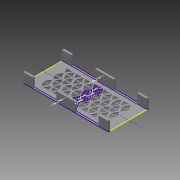
# Autodesk Inventor part: BandSide
Saved by Autodesk Inventor 2014 SP1 (Build 180222100, 222)
## iProperties
Created: 2015-03-16
Part Number: BandSide
Material: Generic
Document SubType Name: Modeling
Designer: Erin
Density: 1 g/cm^3
Appearance: Default
Author: Erin
Autodesk Inventor part; units mm, degrees
ref_plane "YZ Plane" through (0, 0, 0) normal (1, 0, 0) x (0, 1, 0)
ref_plane "XZ Plane" through (0, 0, 0) normal (0, 1, 0) x (-1, 0, 0)
ref_plane "XY Plane" through (0, 0, 0) normal (0, 0, 1) x (1, 0, 0)
sketch "Block1" plane through (0, 0, 0) normal (0, 0, 1) x (1, 0, 0)
  line L0 (-5.6547, 8.5) -> (0.3453, 8.5)
  line L1 (0.3453, 8.5) -> (-2.6547, 3.3038)
  line L2 (-2.6547, 3.3038) -> (-5.6547, 8.5)
  line L3 (5.6547, 3.3038) -> (-0.3453, 3.3038)
  line L4 (-0.3453, 3.3038) -> (2.6547, 8.5)
  line L5 (2.6547, 8.5) -> (5.6547, 3.3038)
  line L6 (-5.6547, 8.5) -> (5.6547, 8.5) construction
  line L7 (5.6547, 8.5) -> (5.6547, 3.3038) construction
  line L8 (5.6547, 3.3038) -> (-5.6547, 3.3038) construction
  line L9 (-5.6547, 3.3038) -> (-5.6547, 8.5) construction
  line L10 (0, 8.5) -> (0, 3.3038) construction
  line L11 (5.6547, 5.9019) -> (-5.6547, 5.9019) construction
  point P0 (0.0717, 5.9721)
  point P1 (-2.6547, 6.7679)
  point P2 (2.6547, 5.0359)
  dimension "d11" = 6
  dimension "d12" = 6
  dimension "d13" = 2
  measures "d11" distance of L0.start L0.end
  measures "d12" distance of L3.start L3.end
  measures "d13" distance between parallel lines of L1 L4
sketch "Sketch1" plane through (0, 0, 0) normal (0, 0, 1) x (1, 0, 0)
  line L0 (-45, 21.5) -> (45, 21.5)
  line L1 (45, 21.5) -> (45, -21.5)
  line L2 (45, -21.5) -> (-45, -21.5)
  line L3 (-45, -21.5) -> (-45, 21.5)
  line L4 (-45, 21.5) -> (-51, 21.5)
  line L5 (-51, 21.5) -> (-51, -21.5)
  line L6 (-51, -21.5) -> (-45, -21.5)
  line L7 (-45, -21.5) -> (-45, 21.5)
  line L8 (-51, 21.5) -> (-91, 21.5)
  line L9 (-91, 21.5) -> (-91, -21.5)
  line L10 (-91, -21.5) -> (-51, -21.5)
  line L11 (-51, -21.5) -> (-51, 21.5)
  line L12 (-91, 21.5) -> (-97, 21.5)
  line L13 (-97, 21.5) -> (-97, -21.5)
  line L14 (-97, -21.5) -> (-91, -21.5)
  line L15 (-91, -21.5) -> (-91, 21.5)
  line L16 (-174.2812, 12.5) -> (-97, 12.5) construction
  line L17 (-97, 12.5) -> (-97, -12.5) construction
  line L18 (-97, -12.5) -> (-174.2812, -12.5) construction
  line L19 (-174.2812, -12.5) -> (-174.2812, 12.5) construction
  line L20 (-127, 31.5284) -> (-127, -21.68) construction
  line L21 (-97, 21.5) -> (-127, 12.5)
  line L22 (-97, -21.5) -> (-127, -12.5)
  line L23 (-127, 12.5) -> (-127, -12.5)
  line L24 (-127, 10) -> (-142, 10)
  line L25 (-142, 10) -> (-142, -10)
  line L26 (-142, -10) -> (-127, -10)
  line L27 (-127, -10) -> (-127, 10)
  point P0 (0, 0)
  point P1 (-45, 0)
  point P2 (0, 21.5)
  point P3 (-97, 0)
  point P4 (-142, 0)
  dimension "d0" = 90
  dimension "d1" = 43
  dimension "d2" = 6
  dimension "d3" = 40
  dimension "d4" = 6
  dimension "d5" = 25
  dimension "d6" = 30
  dimension "d7" = 15
  dimension "d8" = 20
  constraints: 56 end point, 13 parallel, 7 perpendicular, 6 horizontal, 5 point on line, 4 collinear, 4 midpoint, 3 horizontal alignment, 1 vertical alignment
  measures "d0" distance of L1.end L2.end
  measures "d1" distance of L0.end L1.end
  measures "d2" distance of L6.end L5.end
  measures "d3" distance of L10.end L9.end
  measures "d4" distance of L14.end L13.end
  measures "d5" distance of L18.end L16.start
  measures "d6" distance between parallel lines of L20 L13
  measures "d7" distance of L26.end L25.end
  measures "d8" distance of L25.end L24.end
extrude "Extrusion1" add sketch "Sketch1" along normal blind 0.6 contours L0 L1 L2 L3
sketch "Sketch2" plane through (0, 0, 0.6) normal (0, 0, 1) x (1, 0, 0)
  line L0 (-45, 21.5) -> (-45, -21.5) projected
  line L1 (-45, -21.5) -> (45, -21.5) projected
  line L2 (45, -21.5) -> (45, 21.5) projected
  line L3 (45, 21.5) -> (-45, 21.5) projected
  line L4 (-45, -19.5) -> (45, -19.5)
  line L5 (45, 19.5) -> (-45, 19.5)
  line L6 (-45, 19.5) -> (-45, 21.5)
  line L7 (-45, 21.5) -> (45, 21.5)
  line L8 (45, 21.5) -> (45, 19.5)
  line L9 (-45, -19.5) -> (-45, -21.5)
  line L10 (-45, -21.5) -> (45, -21.5)
  line L11 (45, -21.5) -> (45, -19.5)
  line L12 (0, 33.8236) -> (0, -26.1738) construction
  line L13 (-56.1802, 0) -> (59.4276, 0) construction
  line L14 (-5.6547, 14.9904) -> (0.3453, 14.9904)
  line L15 (0.3453, 14.9904) -> (-2.6547, 9.7942)
  line L16 (-2.6547, 9.7942) -> (-5.6547, 14.9904)
  line L17 (5.6547, 9.7942) -> (-0.3453, 9.7942)
  line L18 (-0.3453, 9.7942) -> (2.6547, 14.9904)
  line L19 (2.6547, 14.9904) -> (5.6547, 9.7942)
  line L20 (-5.6547, 14.9904) -> (5.6547, 14.9904) construction
  line L21 (5.6547, 14.9904) -> (5.6547, 9.7942) construction
  line L22 (5.6547, 9.7942) -> (-5.6547, 9.7942) construction
  line L23 (-5.6547, 9.7942) -> (-5.6547, 14.9904) construction
  line L24 (0, 14.9904) -> (0, 9.7942) construction
  line L25 (5.6547, 12.3923) -> (-5.6547, 12.3923) construction
  line L26 (5.6547, 8.7942) -> (-0.3453, 8.7942)
  line L27 (-0.3453, 8.7942) -> (2.6547, 3.5981)
  line L28 (2.6547, 3.5981) -> (5.6547, 8.7942)
  line L29 (-5.6547, 3.5981) -> (0.3453, 3.5981)
  line L30 (0.3453, 3.5981) -> (-2.6547, 8.7942)
  line L31 (-2.6547, 8.7942) -> (-5.6547, 3.5981)
  line L32 (5.6547, 8.7942) -> (-5.6547, 8.7942) construction
  line L33 (-5.6547, 8.7942) -> (-5.6547, 3.5981) construction
  line L34 (-5.6547, 3.5981) -> (5.6547, 3.5981) construction
  line L35 (5.6547, 3.5981) -> (5.6547, 8.7942) construction
  line L36 (0, 8.7942) -> (0, 3.5981) construction
  line L37 (-5.6547, 6.1962) -> (5.6547, 6.1962) construction
  line L38 (-5.6547, 2.5981) -> (0.3453, 2.5981)
  line L39 (0.3453, 2.5981) -> (-2.6547, -2.5981)
  line L40 (-2.6547, -2.5981) -> (-5.6547, 2.5981)
  line L41 (5.6547, -2.5981) -> (-0.3453, -2.5981)
  line L42 (-0.3453, -2.5981) -> (2.6547, 2.5981)
  line L43 (2.6547, 2.5981) -> (5.6547, -2.5981)
  line L44 (-5.6547, 2.5981) -> (5.6547, 2.5981) construction
  line L45 (5.6547, 2.5981) -> (5.6547, -2.5981) construction
  line L46 (5.6547, -2.5981) -> (-5.6547, -2.5981) construction
  line L47 (-5.6547, -2.5981) -> (-5.6547, 2.5981) construction
  line L48 (0, 2.5981) -> (0, -2.5981) construction
  line L49 (5.6547, 0) -> (-5.6547, 0) construction
  line L50 (5.6547, -3.5981) -> (-0.3453, -3.5981)
  line L51 (-0.3453, -3.5981) -> (2.6547, -8.7942)
  line L52 (2.6547, -8.7942) -> (5.6547, -3.5981)
  line L53 (-5.6547, -8.7942) -> (0.3453, -8.7942)
  line L54 (0.3453, -8.7942) -> (-2.6547, -3.5981)
  line L55 (-2.6547, -3.5981) -> (-5.6547, -8.7942)
  line L56 (5.6547, -3.5981) -> (-5.6547, -3.5981) construction
  line L57 (-5.6547, -3.5981) -> (-5.6547, -8.7942) construction
  line L58 (-5.6547, -8.7942) -> (5.6547, -8.7942) construction
  line L59 (5.6547, -8.7942) -> (5.6547, -3.5981) construction
  line L60 (0, -3.5981) -> (0, -8.7942) construction
  line L61 (-5.6547, -6.1962) -> (5.6547, -6.1962) construction
  line L62 (-5.6547, -9.7942) -> (0.3453, -9.7942)
  line L63 (0.3453, -9.7942) -> (-2.6547, -14.9904)
  line L64 (-2.6547, -14.9904) -> (-5.6547, -9.7942)
  line L65 (5.6547, -14.9904) -> (-0.3453, -14.9904)
  line L66 (-0.3453, -14.9904) -> (2.6547, -9.7942)
  line L67 (2.6547, -9.7942) -> (5.6547, -14.9904)
  line L68 (-5.6547, -9.7942) -> (5.6547, -9.7942) construction
  line L69 (5.6547, -9.7942) -> (5.6547, -14.9904) construction
  line L70 (5.6547, -14.9904) -> (-5.6547, -14.9904) construction
  line L71 (-5.6547, -14.9904) -> (-5.6547, -9.7942) construction
  line L72 (0, -9.7942) -> (0, -14.9904) construction
  line L73 (5.6547, -12.3923) -> (-5.6547, -12.3923) construction
  point P0 (0, 0)
  dimension "d17" = 1
  dimension "d18" = 1
  dimension "d19" = 1
  dimension "d21" = 1
  dimension "d14" = 2
  dimension "d15" = 2
  constraints: 20 end point, 6 perpendicular, 6 vertical, 4 point on line, 2 horizontal, 1 collinear, 1 parallel
  measures "d14" distance between parallel lines of L5 L3
  measures "d15" distance between parallel lines of L1 L4
extrude "Extrusion2" cut sketch "Sketch2" against normal blind 5 contours L14 L15 L16 | L17 L18 L19 | L28 L27 L26 | L31 L30 L29 | L38 L39 L40 | L41 L42 L43 | L52 L51 L50 | L55 L54 L53 | L62 L63 L64 | L65 L66 L67
pattern_linear "Rectangular Pattern1" count 4 spacing 10 along (-1, 0, 0) count 4 spacing 10 along (1, 0, 0) of "Extrusion2"
extrude "Extrusion3" add sketch "Sketch2" along normal blind 10 contours L3 L2 L5 L0 | L4 L2 L1 L0
sketch "Sketch3" plane through (-45, 19.5, 0.6) normal (0, -1, 0) x (1, 0, 0)
  line L0 (0, 10) -> (90, 10) projected
  line L1 (0, 0) -> (0, 10) projected
  line L2 (10, 10) -> (35, 10)
  line L3 (35, 10) -> (35, 0)
  line L4 (35, 0) -> (10, 0)
  line L5 (10, 0) -> (10, 10)
  point P0 (45, -0.6)
  dimension "d40" = 25
  dimension "d41" = 10
  dimension "d42" = 10
  constraints: 8 end point, 2 parallel, 1 horizontal, 1 perpendicular, 1 point on line
  measures "d40" distance of L3.end L4.end
  measures "d41" distance of L2.end L3.end
  measures "d42" distance between parallel lines of L1 L5
extrude "Extrusion4" cut sketch "Sketch3" along normal mid plane 100
sketch "Sketch4" plane through (-45, -19.5, 0.6) normal (0, 1, 0) x (1, 0, 0)
  line L0 (90, -10) -> (0, -10) projected
  line L1 (90, 0) -> (90, -10) projected
  line L2 (55, -10) -> (80, -10)
  line L3 (80, -10) -> (80, 0)
  line L4 (80, 0) -> (55, 0)
  line L5 (55, 0) -> (55, -10)
  point P0 (45, 0.6)
  dimension "d43" = 25
  dimension "d44" = 10
  dimension "d45" = 10
  constraints: 8 end point, 2 parallel, 1 horizontal, 1 perpendicular, 1 point on line
  measures "d43" distance of L4.end L3.end
  measures "d44" distance of L3.end L2.end
  measures "d45" distance between parallel lines of L3 L1
extrude "Extrusion5" cut sketch "Sketch4" along normal mid plane 100
body "Solid1"
